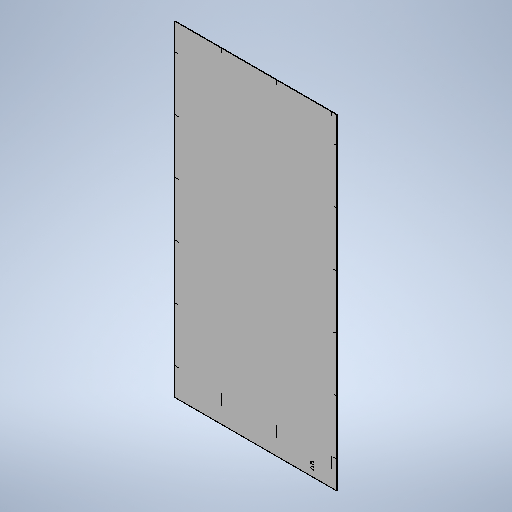
# Autodesk Inventor part: GBK 1211 shield 2
Saved by Autodesk Inventor 2026.2 (Build 302298010, 298A)
## iProperties
Created: 2026-04-17
Part Number: GBK 1211 shield 2
Material: Steel
Document SubType Name: Sheet Metal
Designer: pokla
Density: 7.85 g/cm^3
Sheet Metal Rule: Default_mm
Appearance: Default
Mass: 138487 g
Surface Area: 88564.8 cm^2
Volume: 17641.6 cm^3
Sheet Metal Width: 1480,000 mm
Sheet Metal Length: 2980,000 mm
Sheet Metal Area: 4410400,000 mm^2
Stock Number: 1217
Flat Pattern Width: 148 cm
Flat Pattern Length: 298 cm
Flat Pattern Area: 44104 cm^2
Author: admin
Autodesk Inventor part; units mm, degrees
ref_plane "YZ Plane" through (0, 0, 0) normal (1, 0, 0) x (0, 1, 0)
ref_plane "XZ Plane" through (0, 0, 0) normal (0, 1, 0) x (-1, 0, 0)
ref_plane "XY Plane" through (0, 0, 0) normal (0, 0, 1) x (1, 0, 0)
sketch "Sketch1" plane through (0, 0, 0) normal (0, 0, 1) x (1, 0, 0)
  line L0 (740, -1490) -> (-740, -1490)
  line L1 (-740, -1490) -> (-740, 1490)
  line L2 (-740, 1490) -> (740, 1490)
  line L3 (740, 1490) -> (740, -1490)
  line L4 (740, -1490) -> (-740, 1490) construction
  line L5 (-740, -1490) -> (740, 1490) construction
  point P0 (0, 0)
  dimension "d0" = 1480
  dimension "d1" = 2980
  measures "d0" distance of L1.end L2.end
  measures "d1" distance of L0.end L1.end
extrude "Plate1" add sketch "Sketch1" along normal blind 4
sketch "Sketch4" plane through (0, 0, 4) normal (0, 0, 1) x (1, 0, 0)
  line L0 (770, 1247.3333) -> (710, 1247.3333) projected
  line L1 (770, 750.6667) -> (710, 750.6667) projected
  line L2 (770, 254) -> (710, 254) projected
  line L3 (770, -242.6667) -> (710, -242.6667) projected
  line L4 (770, -739.3333) -> (710, -739.3333) projected
  line L5 (770, -1236) -> (710, -1236) projected
  ellipse E0 centre (690.2486, 1484.5) end of major axis (690.2486, 1514.5) minor radius 0.6803 (690.2486, 1454.5) -> (690.2486, 1514.5) ccw projected
  ellipse E1 centre (-310.0086, 1484.5) end of major axis (-310.0086, 1514.5) minor radius 0.6803 (-310.0086, 1454.5) -> (-310.0086, 1514.5) ccw projected
  line L6 (-710, 1247.3333) -> (-739.3197, 1247.3333) projected
  line L7 (-710, 750.6667) -> (-739.3197, 750.6667) projected
  line L8 (-710, 254) -> (-739.3197, 254) projected
  line L9 (-710, -242.6667) -> (-739.3197, -242.6667) projected
  line L10 (190.12, -1243.5) -> (190.12, -1340.5) projected
  line L11 (-310.0086, -1243.5) -> (-310.0086, -1340.5) projected
  line L12 (690.2486, -1243.5) -> (690.2486, -1340.5) projected
  line L13 (690.2486, -1340.5) -> (686.2496, -1340.5) projected
  line L14 (190.12, -1340.5) -> (186.121, -1340.5) projected
  line L15 (-310.0086, -1340.5) -> (-314.0076, -1340.5) projected
  line L16 (-710, -739.3333) -> (-739.3197, -739.3333) projected
  line L17 (-710, -1236) -> (-739.3197, -1236) projected
  line L18 (690.2486, 1454.5) -> (686.2496, 1454.5) projected
  line L19 (710, 1243.3333) -> (710, 1247.3333) projected
  line L20 (190.12, 1454.5) -> (186.121, 1454.5) projected
  line L21 (-310.0086, 1454.5) -> (-314.0076, 1454.5) projected
  line L22 (-710, 1243.3333) -> (-710, 1247.3333) projected
  line L23 (-710, 746.6667) -> (-710, 750.6667) projected
  line L24 (-710, 250) -> (-710, 254) projected
  line L25 (-710, -743.3333) -> (-710, -739.3333) projected
  line L26 (-710, -1240) -> (-710, -1236) projected
  line L27 (710, -1240) -> (710, -1236) projected
  line L28 (710, -743.3333) -> (710, -739.3333) projected
  line L29 (710, -246.6667) -> (710, -242.6667) projected
  line L30 (710, 250) -> (710, 254) projected
  line L31 (710, 746.6667) -> (710, 750.6667) projected
  ellipse E2 centre (190.12, 1484.5) end of major axis (190.12, 1514.5) minor radius 0.6803 (190.12, 1454.5) -> (190.12, 1514.5) ccw projected
  line L32 (530.9218, -1356.779) -> (530.9218, -1714.4695) construction
  line L33 (530.9218, -1714.4695) -> (479.354, -1714.4695) construction
  line L34 (479.354, -1714.4695) -> (479.354, -1356.779) construction
  line L35 (479.354, -1356.779) -> (530.9218, -1356.779) construction
  line L36 (-710, -246.6667) -> (-710, -242.6667) projected
  point P0 (0, 0)
  constraints: 5 other
mark "Mark2"
equation "\"d0\" = Лист_ширина"
equation "\"d2\" = Thickness"
equation "\"BendRadius\" = Thickness"
equation "\"BendReliefWidth\" = Thickness"
equation "\"BendReliefDepth\" = 0.5 * Thickness"
equation "\"CornerReliefSize\" = 4 * Thickness"
equation "\"MinimumRemnant\" = 2 * Thickness"
equation "\"TransitionRadius\" = BendRadius"
equation "\"JacobiRadiusSize\" = BendRadius"
equation "\"GapSize\" = Thickness"
equation "\"Лист_ширина\" = 1480"
equation "\"Thickness\" = 4"
body "Solid1"
